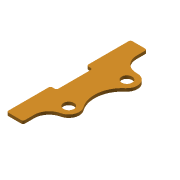
# Autodesk Inventor part: 3136 1133 83
Saved by Autodesk Inventor 2022 Beta2 (Build 260130000, 130) ContinuousBuild 0
## iProperties
Shininess: 64.0
Length Units: 11269
Angle Units: 11279
Time Units: 11290
Mass Units: 11283
Length Display Precision: 3
Angle Display Precision: 2
Compacted: True
Part Number: 3136 1133 83
Document SubType Name: Modeling
Created: 2003-04-13
Designer: Uffe Bak
Material: Steel, Mild
Density: 7.86 g/cm^3
Appearance: Brokk-Gul
Density: 0.0
Volumn: 0.0
Area: 0.0
PropertySet Name: Model Information
Control State: 0
Master: False
Checked Out: False
Author: Uffe Bak
Autodesk Inventor part; units mm, degrees
ref_plane "YZ Plane" through (0, 0, 0) normal (1, 0, 0) x (0, 1, 0)
ref_plane "XZ Plane" through (0, 0, 0) normal (0, 1, 0) x (-1, 0, 0)
ref_plane "XY Plane" through (0, 0, 0) normal (0, 0, 1) x (1, 0, 0)
sketch "Sketch1" plane through (0, 0, 0) normal (0, 0, 1) x (0, 1, 0)
  line L0 (98.3739, 70.6898) -> (232.7239, 70.6898)
  line L1 (238.7239, 64.6898) -> (238.7239, 56.6898)
  line L2 (244.7239, 50.6898) -> (352.7239, 50.6898)
  line L3 (358.7239, 56.6898) -> (358.7239, 64.6898)
  line L4 (364.7239, 70.6898) -> (499.0739, 70.6898)
  line L5 (505.0739, 64.6898) -> (505.0739, 21.6898)
  line L6 (499.0739, 15.6898) -> (470.0209, 15.6898)
  arc A0 (470.0209, 15.6898) -> (420.0521, -36.0749) centre (470.0209, -34.3102) ccw
  arc A1 (358.3704, -59.936) -> (420.0521, -36.0749) centre (385.0739, -37.3102) ccw
  arc A2 (358.3704, -59.936) -> (232.9093, -44.7528) centre (287.4489, -120.0273) ccw
  arc A3 (178.1588, -23.7808) -> (232.9093, -44.7528) centre (212.3739, -16.4102) ccw
  line L7 (129.28, 15.6898) -> (98.3739, 15.6898)
  line L8 (92.3739, 21.6898) -> (92.3739, 64.6898)
  circle A4 centre (212.3739, -16.4102) radius 17.5
  circle A5 centre (385.0739, -37.3102) radius 17.5
  arc A6 (178.1588, -23.7808) -> (129.28, 15.6898) centre (129.28, -34.3102) ccw
  arc A7 (92.3739, 21.6898) -> (98.3739, 15.6898) centre (98.3739, 21.6898) ccw
  arc A8 (98.3739, 70.6898) -> (92.3739, 64.6898) centre (98.3739, 64.6898) ccw
  arc A9 (238.7239, 64.6898) -> (232.7239, 70.6898) centre (232.7239, 64.6898) ccw
  arc A10 (238.7239, 56.6898) -> (244.7239, 50.6898) centre (244.7239, 56.6898) ccw
  arc A11 (352.7239, 50.6898) -> (358.7239, 56.6898) centre (352.7239, 56.6898) ccw
  arc A12 (364.7239, 70.6898) -> (358.7239, 64.6898) centre (364.7239, 64.6898) ccw
  arc A13 (505.0739, 64.6898) -> (499.0739, 70.6898) centre (499.0739, 64.6898) ccw
  arc A14 (499.0739, 15.6898) -> (505.0739, 21.6898) centre (499.0739, 21.6898) ccw
  point P0 (238.7239, 50.6898)
  point P1 (358.7239, 50.6898)
  point P2 (505.0739, 70.6898)
  point P3 (505.0739, 15.6898)
  dimension "d0" = 172.7
  dimension "d1" = 20.9
  dimension "d2" = 67.1
  dimension "d3" = 20
  dimension "d4" = 35
  dimension "d5" = 35
  dimension "d6" = 120
  dimension "d7" = 120
  dimension "d8" = 120
  dimension "d9" = 55
  dimension "d10" = 35
  dimension "d11" = 35
  dimension "d12" = 50
  dimension "d13" = 50
  dimension "d14" = 26.35
  dimension "d15" = 6
  constraints: 26 point on circle, 22 tangent, 18 end point, 15 centre point, 8 point on line, 7 equal radius, 6 parallel, 3 collinear, 2 coincident, 2 concentric, 1 horizontal, 1 perpendicular
  measures "d0" horizontal distance of A1.centre A3.centre
  measures "d1" vertical distance of A1.centre A3.centre
  measures "d2" distance from line of L2 A3.centre
  measures "d3" distance between parallel lines of L0 L2
  measures "d4" diameter of A4
  measures "d5" diameter of A5
  measures "d6" distance of point (238.724, 50.69) point (358.724, 50.69)
  measures "d7" distance from line of L5 A1.centre
  measures "d8" distance from line of L8 A3.centre
  measures "d9" distance of point (505.074, 70.69) point (505.074, 15.69)
  measures "d10" radius of A3
  measures "d11" radius of A1
  measures "d12" radius of A0
  measures "d13" radius of A6
  measures "d14" distance from line of L1 A3.centre
  measures "d15" radius of A7
extrude "Extrusion1" add sketch "Sketch1" along normal blind 10
equation "\"d14\" = -0.5 * d6 + 0.5 * d0"
body "Solid1"
